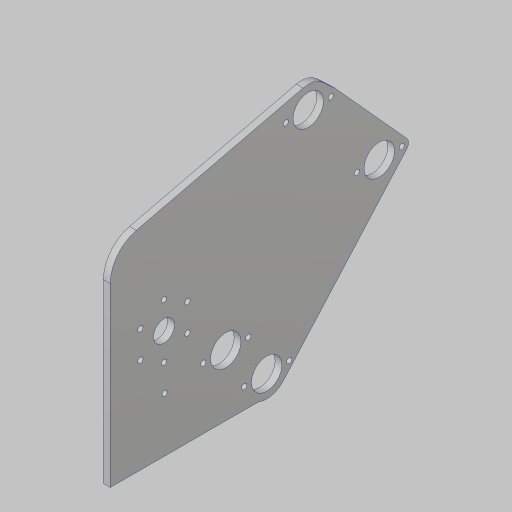
# Autodesk Inventor part: GI - 001
Saved by Autodesk Inventor 2023.5 (Build 275446000, 446)
## iProperties
Created: 2025-01-17
Part Number: GI - 001
Material: Aluminum 6061
Document SubType Name: Modeling
Designer: mavericks
Density: 2.7 g/cm^3
Appearance: Aluminum - Flat
Author: mavericks
Autodesk Inventor part; units mm, degrees
ref_plane "YZ Plane" through (0, 0, 0) normal (1, 0, 0) x (0, 1, 0)
ref_plane "XZ Plane" through (0, 0, 0) normal (0, 1, 0) x (-1, 0, 0)
ref_plane "XY Plane" through (0, 0, 0) normal (0, 0, 1) x (1, 0, 0)
sketch "Sketch2" plane through (0, 0, 0) normal (1, 0, 0) x (0, 1, 0)
  line L0 (63.5, 38.1) -> (-63.5, 38.1) construction
  line L1 (-63.5, 38.1) -> (-63.5, -38.1) construction
  line L2 (-63.5, -38.1) -> (63.5, -38.1) construction
  line L3 (63.5, -38.1) -> (63.5, 38.1) construction
  line L4 (63.5, 38.1) -> (-63.5, -38.1) construction
  line L5 (-63.5, 38.1) -> (63.5, -38.1) construction
  line L6 (-63.5, 38.1) -> (-76.2, 38.1) construction
  line L7 (-76.2, 38.1) -> (-76.2, -266.7) construction
  line L8 (-76.2, -266.7) -> (-63.5, -266.7) construction
  line L9 (-63.5, -266.7) -> (-63.5, 38.1) construction
  circle A0 centre (24.3307, -140.8335) radius 57.15 construction
  circle A1 centre (-50.8, -108.1179) radius 15.875 construction
  circle A2 centre (-12.7, -69.85) radius 25.4 construction
  circle A3 centre (69.85, -213.36) radius 38.1 construction
  circle A4 centre (69.85, -213.36) radius 14.2875
  circle A5 centre (143.2804, -146.9613) radius 38.1 construction
  circle A6 centre (143.2804, -146.9613) radius 14.2875
  circle A7 centre (-50.8, -108.1179) radius 14.2875
  circle A8 centre (-12.7, -69.85) radius 14.2875
  line L10 (-69.85, 38.1) -> (-69.85, -100.1804)
  line L11 (-69.85, 38.1) -> (95.25, 38.1)
  line L12 (126.1319, 13.7236) -> (163.3537, -142.1685)
  arc A9 (126.1319, 13.7236) -> (95.25, 38.1) centre (95.25, 6.35) ccw
  line L13 (-57.15, 38.1) -> (-6.35, 38.1) construction
  line L14 (-6.35, 38.1) -> (-6.35, 444.5) construction
  line L15 (-6.35, 444.5) -> (-57.15, 444.5) construction
  line L16 (-57.15, 444.5) -> (-57.15, 38.1) construction
  line L17 (143.2804, -167.9798) -> (143.2804, -125.9428) construction
  line L18 (69.85, -192.3415) -> (69.85, -234.3785) construction
  line L19 (-12.7, -48.8315) -> (-12.7, -90.8685) construction
  line L20 (-50.8, -87.0994) -> (-50.8, -129.1364) construction
  circle A10 centre (69.85, -234.3785) radius 6.35 construction
  circle A11 centre (69.85, -213.36) radius 20.6375 construction
  circle A12 centre (143.2804, -146.9613) radius 20.6375 construction
  circle A13 centre (-50.8, -108.1179) radius 20.6375 construction
  circle A14 centre (143.2804, -167.9798) radius 6.35 construction
  line L21 (147.5394, -172.6898) -> (74.1089, -239.0885)
  line L22 (-64.5042, -123.5485) -> (65.6333, -239.1264)
  arc A15 (-69.85, -100.1804) -> (-64.5042, -123.5485) centre (-50.8, -108.1179) ccw
  arc A16 (65.6333, -239.1264) -> (74.1089, -239.0885) centre (69.85, -234.3785) ccw
  arc A17 (158.4167, -160.9899) -> (163.3537, -142.1685) centre (143.2804, -146.9613) ccw
  line L23 (158.4167, -160.9899) -> (147.9378, -172.2963)
  arc A18 (147.5394, -172.6898) -> (147.9378, -172.2963) centre (143.2804, -167.9798) ccw
  point P0 (0, 0)
  point P1 (-14.3002, 165.1)
  point P2 (-49.1998, 165.1)
  point P3 (-14.3002, 190.5)
  point P4 (-49.1998, 190.5)
  point P5 (-14.3002, 215.9)
  point P6 (-49.1998, 215.9)
  point P7 (-14.3002, 241.3)
  point P8 (-49.1998, 241.3)
  dimension "d2" = 127
  dimension "d3" = 76.2
  dimension "d4" = 12.7
  dimension "d5" = 304.8
  dimension "d6" = 114.3
  dimension "d7" = 31.75
  dimension "d8" = 50.8
  dimension "d9" = 76.2
  dimension "d10" = 146.05
  dimension "d11" = 28.575
  dimension "d12" = 31.75
  dimension "d13" = 25.4
  dimension "d14" = 54.0004
  dimension "d15" = 50.8
  dimension "d16" = 175.26
  dimension "d17" = 76.2
  dimension "d18" = 98.999
  dimension "d20" = 28.575
  dimension "d21" = 28.575
  dimension "d22" = 28.575
  dimension "d28" = 165.1
  dimension "d30" = 31.75
  dimension "d40" = 50.8
  dimension "d41" = 19.05
  dimension "d42" = 406.4
  dimension "d43" = 127
  dimension "d44" = 7.9502
  dimension "d45" = 7.9502
  dimension "d48" = 25.4
  dimension "d70" = 174.0002
  dimension "d80" = 42.037
  dimension "d81" = 42.037
  dimension "d82" = 42.037
  dimension "d83" = 42.037
  dimension "d84" = 12.7
  dimension "d85" = 6.35
  dimension "d86" = 6.35
  dimension "d87" = 6.35
  dimension "d88" = 12.7
  constraints: 48 end point, 19 centre point, 18 point on circle, 14 coincident, 10 tangent, 7 midpoint, 6 parallel, 5 vertical, 4 perpendicular, 3 horizontal, 1 concentric, 1 horizontal alignment, 1 point on line, 6 other
  measures "d2" distance of L2.end L1.end
  measures "d3" distance of L1.end L0.end
  measures "d4" distance of L8.end L7.end
  measures "d5" distance of L7.end L6.end
  measures "d6" diameter of A0
  measures "d7" diameter of A1
  measures "d8" diameter of A2
  measures "d9" diameter of A3
  measures "d10" distance from line of A3.centre L7
  measures "d11" diameter of A4
  measures "d12" distance from line of A2.centre L2
  measures "d13" distance from line of L7 A1.centre
  measures "d14" distance of A2.centre A1.centre
  measures "d15" distance from line of L9 A2.centre
  measures "d16" distance from line of L2 A3.centre
  measures "d17" diameter of A5
  measures "d18" distance of A3.centre A5.centre
  measures "d20" diameter of A6
  measures "d21" diameter of A7
  measures "d22" diameter of A8
  measures "d28" distance of L11.end L10.start
  measures "d30" radius of A9
  measures "d40" distance of L15.end L14.end
  measures "d41" distance between parallel lines of L16 L7
  measures "d42" distance of L15.end L13.start
  measures "d43" distance from line of L0 point (-14.3, 165.1)
  measures "d44" distance from line of L14 point (-14.3, 165.1)
  measures "d45" distance from line of L16 point (-49.2, 165.1)
  measures "d48" distance of point (-14.3, 165.1) point (-14.3, 190.5)
  measures "d70" distance of A2.centre A5.centre
  measures "d80" distance of L17.start L17.end
  measures "d81" distance of L18.start L18.end
  measures "d82" distance of L19.start L19.end
  measures "d83" distance of L20.start L20.end
  measures "d84" diameter of A10
  measures "d85" radial gap between concentric circles of A4 A11
  measures "d86" radial gap between concentric circles of A6 A12
  measures "d87" radial gap between concentric circles of A7 A13
  measures "d88" diameter of A14
extrude "Extrusion1" add sketch "Sketch2" along normal blind 6.35
sketch "Sketch3" plane through (6.35, 0, 0) normal (1, 0, 0) x (0, 0, -1)
  line L0 (-38.1, 63.5) -> (38.1, 63.5) construction
  line L1 (38.1, 63.5) -> (38.1, -63.5) construction
  line L2 (38.1, -63.5) -> (-38.1, -63.5) construction
  line L3 (-38.1, -63.5) -> (-38.1, 63.5) construction
  line L4 (-38.1, 63.5) -> (38.1, -63.5) construction
  line L5 (38.1, 63.5) -> (-38.1, -63.5) construction
  line L6 (-38.1, -69.85) -> (100.1804, -69.85) construction
  line L7 (-38.1, 95.25) -> (-38.1, -69.85) construction
  point P0 (0, 0)
  point P1 (0, 0)
  dimension "d36" = 76.2
  dimension "d37" = 127
  dimension "d38" = 6.35
  dimension "d39" = 0
  constraints: 12 end point, 2 midpoint, 2 parallel, 1 horizontal, 1 perpendicular
  measures "d36" distance of L1.end L2.end
  measures "d37" distance of L0.end L1.end
  measures "d38" distance between parallel lines of L6 L2
  measures "d39" distance between parallel lines of L7 L3
sketch "Sketch4" plane through (0, 0, 0) normal (-1, 0, 0) x (0, 0, 1)
  circle A0 centre (-12.1007, 31.75) radius 9.906
  circle A1 centre (-213.36, 69.85) radius 14.2875 projected
  circle A2 centre (-146.9613, 143.2804) radius 14.2875 projected
  circle A3 centre (-108.1179, -50.8) radius 14.2875 projected
  circle A4 centre (-69.85, -12.7) radius 14.2875 projected
  arc A5 (38.1, 95.25) -> (13.7236, 126.1319) centre (6.35, 95.25) ccw projected
  line L0 (38.1, 95.25) -> (38.1, -69.85) projected
  line L1 (38.1, -69.85) -> (-100.1804, -69.85) projected
  line L2 (-142.1685, 163.3537) -> (13.7236, 126.1319) projected
  circle A6 centre (-213.36, 69.85) radius 14.2875 projected
  circle A7 centre (-146.9613, 143.2804) radius 14.2875 projected
  circle A8 centre (-108.1179, -50.8) radius 14.2875 projected
  circle A9 centre (-69.85, -12.7) radius 14.2875 projected
  line L3 (38.1, 95.25) -> (38.1, -69.85) projected
  line L4 (38.1, -69.85) -> (-100.1804, -69.85) projected
  circle A10 centre (-12.1007, 31.75) radius 25.4 construction
  arc A11 (38.1, 95.25) -> (13.7236, 126.1319) centre (6.35, 95.25) ccw projected
  line L5 (-142.1685, 163.3537) -> (13.7236, 126.1319) projected
  arc A12 (-123.5485, -64.5042) -> (-100.1804, -69.85) centre (-108.1179, -50.8) ccw projected
  line L6 (-123.5485, -64.5042) -> (-239.1264, 65.6333) projected
  arc A13 (-239.0885, 74.1089) -> (-239.1264, 65.6333) centre (-234.3785, 69.85) ccw projected
  line L7 (-239.0885, 74.1089) -> (-172.6898, 147.5394) projected
  arc A14 (-123.5485, -64.5042) -> (-100.1804, -69.85) centre (-108.1179, -50.8) ccw projected
  line L8 (-123.5485, -64.5042) -> (-239.1264, 65.6333) projected
  arc A15 (-239.0885, 74.1089) -> (-239.1264, 65.6333) centre (-234.3785, 69.85) ccw projected
  line L9 (-239.0885, 74.1089) -> (-172.6898, 147.5394) projected
  arc A16 (-172.2963, 147.9378) -> (-172.6898, 147.5394) centre (-167.9798, 143.2804) ccw projected
  line L10 (-172.2963, 147.9378) -> (-160.9899, 158.4167) projected
  arc A17 (-142.1685, 163.3537) -> (-160.9899, 158.4167) centre (-146.9613, 143.2804) ccw projected
  arc A18 (-172.2963, 147.9378) -> (-172.6898, 147.5394) centre (-167.9798, 143.2804) ccw projected
  line L11 (-172.2963, 147.9378) -> (-160.9899, 158.4167) projected
  arc A19 (-142.1685, 163.3537) -> (-160.9899, 158.4167) centre (-146.9613, 143.2804) ccw projected
  point P0 (0, 0)
  point P1 (-12.1007, 57.15)
  point P2 (-34.0977, 44.45)
  point P3 (-34.0977, 19.05)
  point P4 (-12.1007, 6.35)
  point P5 (9.8964, 19.05)
  point P6 (9.8964, 44.45)
  dimension "d58" = 50.8
  dimension "d53" = 19.812
  dimension "d54" = 72.8751
  dimension "d55" = 101.6
  dimension "d61" = 360
  constraints: 2 vertical alignment, 1 centre point, 1 coincident, 9 other
  measures "d53" diameter of A0
  measures "d54" distance of A0.centre A4.centre
  measures "d55" distance from line of L1 A0.centre
extrude "Extrusion2" cut sketch "Sketch4" against normal blind 25.4 contours A0
hole "Hole1" at (0, 57.15, -12.1007) at (0, 44.45, -34.0977) at (0, 19.05, -34.0977) at (0, 6.35, -12.1007) at (0, 19.05, 9.8964) at (0, 44.45, 9.8964) direction (1, 0, 0) diameter 5.1054 end through all clearance for "Flat Head Machine Screw (82)" size "#10" standard "Ansi Unified Screw Threads"
sketch "Sketch5" plane through (6.35, 0, 0) normal (1, 0, 0) x (0, 0, -1)
  line L0 (-38.1, 95.25) -> (-38.1, -69.85) projected
  line L1 (-38.1, -69.85) -> (100.1804, -69.85) projected
  point P0 (0, 0)
  point P1 (12.7, -19.05)
  dimension "d71" = 50.8
  dimension "d72" = 50.8
  measures "d71" distance from line of L0 point (12.7, -19.05)
  measures "d72" distance from line of L1 point (12.7, -19.05)
hole "Hole2" at (6.35, -19.05, -12.7) direction (-1, 0, 0) diameter 5.1054 end through all clearance for "Flat Head Machine Screw (82)" size "#10" standard "Ansi Unified Screw Threads"
hole "Hole3" at (0, -14.3002, 165.1) at (0, -49.1998, 165.1) at (0, -14.3002, 190.5) at (0, -49.1998, 190.5) at (0, -14.3002, 215.9) at (0, -49.1998, 215.9) at (0, -14.3002, 241.3) at (0, -49.1998, 241.3) at (0, 143.2804, -167.9798) at (0, 143.2804, -125.9428) at (0, 69.85, -192.3415) at (0, 69.85, -234.3785) at (0, -12.7, -48.8315) at (0, -12.7, -90.8685) at (0, -50.8, -87.0994) at (0, -50.8, -129.1364) direction (1, 0, 0) diameter 5.1054 end through all clearance for "Flat Head Machine Screw (82)" size "#10" standard "Ansi Unified Screw Threads"
body "Solid1"
